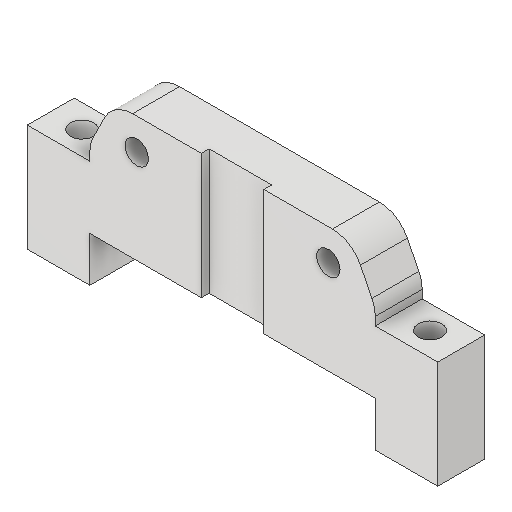
# Autodesk Inventor part: 3DP_ABS_Electromagnet_Clamps
Saved by Autodesk Inventor 2026.1 (Build 301233000, 233)
## iProperties
Created: 2018-05-26
Part Number: 3DP_ABS_Electromagnet_Clamps
Material: ABS Plastic
Document SubType Name: Modeling
Designer: Andrzej
Density: 1.06 g/cm^3
Appearance: Smooth - White
Author: Andrzej
Autodesk Inventor part; units mm, degrees
ref_plane "YZ Plane" through (0, 0, 0) normal (1, 0, 0) x (0, 1, 0)
ref_plane "XZ Plane" through (0, 0, 0) normal (0, 1, 0) x (-1, 0, 0)
ref_plane "XY Plane" through (0, 0, 0) normal (0, 0, 1) x (1, 0, 0)
sketch "Sketch1" plane through (0, 0, 0) normal (0, 0, 1) x (1, 0, 0)
  line L0 (-18.25, 6.5) -> (18.25, 6.5)
  line L1 (18.25, 6.5) -> (18.25, -6.5)
  line L2 (18.25, -6.5) -> (-18.25, -6.5)
  line L3 (-18.25, -6.5) -> (-18.25, 6.5)
  line L4 (26.25, 14.5) -> (-26.25, 14.5)
  line L5 (-26.25, 14.5) -> (-26.25, -14.5)
  line L6 (-26.25, -14.5) -> (26.25, -14.5)
  line L7 (26.25, -14.5) -> (26.25, 14.5)
  line L8 (-26.25, 0.75) -> (-18.25, 0.75)
  line L9 (18.25, 0.75) -> (26.25, 0.75)
  point P0 (0, 0)
  dimension "d0" = 36.5
  dimension "d1" = 13
  dimension "d2" = 8
  dimension "d3" = 18.25
  dimension "d4" = 6.5
  dimension "d5" = 0.75
  dimension "d6" = 0.75
  constraints: 20 end point, 4 parallel, 4 perpendicular, 4 point on line, 1 horizontal, 3 other
  measures "d0" distance of L1.end L2.end
  measures "d1" distance of L0.end L1.end
  measures "d2" distance between parallel lines of L0 L4
  measures "d3" distance from line of L3 point (0, 0)
  measures "d4" distance from line of L0 point (0, 0)
  measures "d5" distance from line of point (0, 0) L8
  measures "d6" distance from line of point (0, 0) L9
extrude "Extrusion1" add sketch "Sketch1" along normal blind 6 contours L3 L8 L5 L4 L7 L9 L1 L0
sketch "Sketch2" plane through (18.25, 0.75, 0) normal (0, -1, 0) x (1, 0, 0)
  line L0 (-44.5, 0) -> (-36.5, 0) projected
  line L1 (-36.5, 0) -> (-36.5, 6) projected
  line L2 (-44.5, 6) -> (-36.5, 6) projected
  line L3 (-44.5, 0) -> (-44.5, 6) projected
  line L4 (0, 0) -> (8, 0) projected
  line L5 (8, 0) -> (8, 6) projected
  line L6 (0, 6) -> (8, 6) projected
  line L7 (0, 0) -> (0, 6) projected
  point P0 (-18.25, 0)
  point P1 (-40.5, 3)
  point P2 (4, 3)
  dimension "d9" = 8
  dimension "d10" = 6
  dimension "d11" = 3
  dimension "d12" = 4
  dimension "d13" = 4
  dimension "d14" = 3
  measures "d9" distance of L2.start L1.end
  measures "d10" distance of L0.start L2.start
  measures "d11" distance from line of L2 point (-40.5, 3)
  measures "d12" distance from line of L1 point (-40.5, 3)
  measures "d13" distance from line of L5 point (4, 3)
  measures "d14" distance from line of L6 point (4, 3)
hole "Hole1" at (-22.25, 0.75, 3) at (22.25, 0.75, 3) direction (0, 1, 0) diameter 3 end through all
sketch "Sketch3" plane through (0, 0, 0) normal (0, 0, -1) x (-1, 0, 0)
  line L0 (18.25, 6.5) -> (-18.25, 6.5) projected
  line L1 (18.25, 0.75) -> (18.25, 6.5) projected
  line L2 (26.25, 0.75) -> (18.25, 0.75) projected
  line L3 (26.25, 14.5) -> (26.25, 0.75) projected
  line L4 (-26.25, 14.5) -> (26.25, 14.5) projected
  line L5 (-26.25, 0.75) -> (-26.25, 14.5) projected
  line L6 (-18.25, 0.75) -> (-26.25, 0.75) projected
  line L7 (-18.25, 6.5) -> (-18.25, 0.75) projected
  line L8 (-26.25, 14.5) -> (26.25, 14.5) projected
  line L9 (18.25, 14.5) -> (-18.25, 14.5)
  line L10 (-18.25, 14.5) -> (-18.25, 22.5)
  line L11 (-18.25, 22.5) -> (18.25, 22.5)
  line L12 (18.25, 22.5) -> (18.25, 14.5)
  point P0 (0, 0)
  point P1 (12.25, 18.5)
  point P2 (-12.25, 18.5)
  dimension "d22" = 36.5
  dimension "d23" = 8
  dimension "d24" = 8
  dimension "d25" = 6
  dimension "d26" = 6
  dimension "d27" = 4
  dimension "d28" = 4
  constraints: 8 end point, 2 parallel, 1 horizontal, 1 perpendicular, 1 point on line
  measures "d22" distance between parallel lines of L10 L12
  measures "d23" distance between parallel lines of L3 L12
  measures "d24" distance between parallel lines of L4 L11
  measures "d25" distance from line of L12 point (12.25, 18.5)
  measures "d26" distance from line of L10 point (-12.25, 18.5)
  measures "d27" distance from line of point (12.25, 18.5) L11
  measures "d28" distance from line of L11 point (-12.25, 18.5)
extrude "Extrusion2" add sketch "Sketch3" against normal blind 6 contours L4 L10 L11 L12
hole "Hole2" at (-12.25, 18.5, 0) at (12.25, 18.5, 0) direction (0, 0, 1) diameter 3 end through all
chamfer "Chamfer1" distance 3 distance2 6 1 edges at (-18.25, 22.5, 3) measured on face at (-6.0833, 22.5, 2)
chamfer "Chamfer2" distance 3 distance2 6 1 edges at (18.25, 22.5, 3) measured on face at (-4.0833, 22.5, 2)
fillet "Fillet1" radius 4 4 edges at (18.25, 16.5, 3) (15.25, 22.5, 3) (-15.25, 22.5, 3) (-18.25, 16.5, 3)
sketch "Sketch4" plane through (0, 0, 6) normal (0, 0, 1) x (1, 0, 0)
  circle A0 centre (12.25, 18.5) radius 1.5 projected
  circle A1 centre (-12.25, 18.5) radius 1.5 projected
  arc A2 (-17.8277, 17.3446) -> (-18.25, 15.5557) centre (-14.25, 15.5557) ccw projected
  line L0 (-18.25, 15.5557) -> (-18.25, 14.5) projected
  line L1 (-18.25, 14.5) -> (-26.25, 14.5) projected
  line L2 (-26.25, 14.5) -> (-26.25, 0.75) projected
  line L3 (-26.25, 0.75) -> (-18.25, 0.75) projected
  line L4 (-18.25, 0.75) -> (-18.25, 6.5) projected
  line L5 (-18.25, 6.5) -> (18.25, 6.5) projected
  line L6 (18.25, 6.5) -> (18.25, 0.75) projected
  line L7 (18.25, 0.75) -> (26.25, 0.75) projected
  line L8 (26.25, 0.75) -> (26.25, 14.5) projected
  line L9 (26.25, 14.5) -> (18.25, 14.5) projected
  line L10 (18.25, 14.5) -> (18.25, 15.5557) projected
  arc A3 (18.25, 15.5557) -> (17.8277, 17.3446) centre (14.25, 15.5557) ccw projected
  line L11 (16.3556, 20.2889) -> (17.8277, 17.3446) projected
  arc A4 (16.3556, 20.2889) -> (12.7779, 22.5) centre (12.7779, 18.5) ccw projected
  line L12 (12.7779, 22.5) -> (-12.7779, 22.5) projected
  arc A5 (-12.7779, 22.5) -> (-16.3556, 20.2889) centre (-12.7779, 18.5) ccw projected
  line L13 (-17.8277, 17.3446) -> (-16.3556, 20.2889) projected
  line L14 (-18.25, 6.5) -> (18.25, 6.5) projected
  line L15 (-4, 6.5) -> (4, 6.5)
  line L16 (4, 6.5) -> (4, 22.5)
  line L17 (4, 22.5) -> (-4, 22.5)
  line L18 (-4, 22.5) -> (-4, 6.5)
  point P0 (0, 0)
  dimension "d45" = 8
  dimension "d46" = 16
  dimension "d47" = 36.5
  dimension "d48" = 14.25
  dimension "d51" = 16
  constraints: 8 end point, 2 parallel, 1 horizontal, 1 perpendicular, 1 point on line
  measures "d45" distance of L17.end L16.end
  measures "d46" distance of L16.end L15.end
  measures "d47" distance of L4.end L5.end
  measures "d48" distance between parallel lines of L4 L18
  measures "d51" distance between parallel lines of L12 L5
extrude "Extrusion3" cut sketch "Sketch4" against normal blind 1 contours L12 L16 L5 L18
equation "\"d3\" = 0.5 * d0"
equation "\"d4\" = 0.5 * d1"
equation "\"d6\" = d5"
equation "\"d11\" = 0.5 * d10"
equation "\"d12\" = 0.5 * d9"
equation "\"d13\" = d12"
equation "\"d14\" = d11"
equation "\"d27\" = 0.5 * d24"
equation "\"d28\" = d27"
equation "\"d46\" = d51"
equation "\"d48\" = -0.5 * d45 + 0.5 * d47"
body "Solid1"
